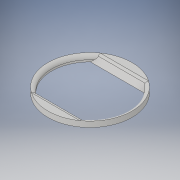
# Autodesk Inventor part: limit_cone
Saved by Autodesk Inventor 2019 (Build 230136000, 136)
## iProperties
Created: 2019-05-25
Part Number: limit_cone
Material: Generic
Document SubType Name: Modeling
Designer: assman
Density: 1 g/cm^3
Appearance: Default
Author: assman
## iProperties of the stored document limit_cone_3DPrint.ipt
Created: 2019-05-25
Part Number: limit_cone_3DPrint
Material: Generic
Document SubType Name: Modeling
Designer: assman
Density: 1 g/cm^3
Appearance: Default
Author: assman
Autodesk Inventor part; units mm, degrees
ref_plane "YZ Plane" through (0, 0, 0) normal (1, 0, 0) x (0, 1, 0)
ref_plane "XZ Plane" through (0, 0, 0) normal (0, 1, 0) x (-1, 0, 0)
ref_plane "XY Plane" through (0, 0, 0) normal (0, 0, 1) x (1, 0, 0)
sketch "Sketch1" plane through (0, 0, 0) normal (0, 1, 0) x (-1, 0, 0)
  circle A0 centre (0, 0) radius 22.85
  circle A1 centre (0, 0) radius 20.85
  dimension "d0" = 45.7
  dimension "d1" = 2
  constraints: 2 centre point, 1 coincident
  measures "d0" diameter of A0
  measures "d1" radial gap between concentric circles of A0 A1
extrude "Extrusion1" add sketch "Sketch1" along normal blind 3
sketch "Sketch2" plane through (0, 3, 0) normal (0, 1, 0) x (1, 0, 0)
  circle A0 centre (0, 0) radius 22.85 construction
  circle A1 centre (0, 0) radius 20.85 construction
  circle A2 centre (0, 0) radius 22.85 construction
  line L0 (14.6356, -14.85) -> (-14.6356, -14.85)
  line L1 (14.6356, 14.85) -> (-14.6356, 14.85)
  arc A3 (-14.6356, -14.85) -> (14.6356, -14.85) centre (0, 0) ccw
  arc A4 (14.6356, 14.85) -> (-14.6356, 14.85) centre (0, 0) ccw
  dimension "d4" = 8
  dimension "d5" = 8
  constraints: 8 point on circle, 4 end point, 2 centre point, 2 coincident, 2 horizontal
  measures "d4" distance edge to line of A0 L0
  measures "d5" distance edge to line of A0 L1
extrude "Extrusion2" add sketch "Sketch2" against normal blind 3
chamfer "Chamfer1" distance 3 angle 45 2 edges at (0, 3, 14.85) (0, 3, -14.85)
fillet "Fillet1" radius 2 6 edges at (0, 3, 17.8499) (12.7936, 3, 16.4635) (12.7936, 3, -16.4635) (-12.7936, 3, 16.4635) (-12.7936, 3, -16.4635) (0, 3, -17.8499)
body "Solid1"
